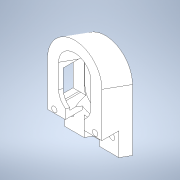
# Autodesk Inventor part: Hauptschalter
Saved by Autodesk Inventor 2021 (Build 250183000, 183)
## iProperties
Created: 2024-06-23
Part Number: Hauptschalter
Material: Generic
Document SubType Name: Modeling
Designer: Lukas
Density: 1 g/cm^3
Appearance: Default
Author: Lukas
Autodesk Inventor part; units mm, degrees
ref_plane "YZ Plane" through (0, 0, 0) normal (1, 0, 0) x (0, 1, 0)
ref_plane "XZ Plane" through (0, 0, 0) normal (0, 1, 0) x (-1, 0, 0)
ref_plane "XY Plane" through (0, 0, 0) normal (0, 0, 1) x (1, 0, 0)
sketch "Sketch1" plane through (0, 0, 0) normal (0, 0, 1) x (1, 0, 0)
  line L0 (-16, 37.209) -> (-16, 0)
  line L1 (-16, 0) -> (16, 0)
  line L2 (16, 0) -> (16, 37.209)
  arc A0 (16, 37.209) -> (-16, 37.209) centre (0, 37.209) ccw
  arc A1 (9.5, 37.209) -> (-9.5, 37.209) centre (0, 37.209) ccw
  arc A2 (-9.5, 23.375) -> (9.5, 23.375) centre (0, 23.375) ccw
  line L3 (-9.5, 23.375) -> (-9.5, 37.209)
  line L4 (9.5, 37.209) -> (9.5, 23.375)
  circle A3 centre (12, 11.493) radius 1.6
  circle A4 centre (-12, 11.493) radius 1.6
  circle A5 centre (0, 48.493) radius 1.6
  line L5 (-5, 45.2867) -> (-5, 41.2867)
  line L6 (-5, 41.2867) -> (5, 41.2867)
  line L7 (5, 41.2867) -> (5, 45.2867)
  line L8 (16, 37.209) -> (16, 53.209)
  line L9 (16, 53.209) -> (-16, 53.209)
  line L10 (-16, 53.209) -> (-16, 37.209)
  circle A6 centre (12, 18.493) radius 1.6
  circle A7 centre (-12, 18.493) radius 1.6
  point P0 (0, 0)
  point P1 (0, 0)
  point P2 (16, 18.6045)
  point P3 (0, 53.209)
  dimension "d0" = 32
  dimension "d1" = 37.209
  dimension "d2" = 13.834
  dimension "d3" = 19
  dimension "d5" = 12
  dimension "d6" = 12
  dimension "d8" = 3.2
  dimension "d26" = 10
  dimension "d27" = 4
  dimension "d34" = 37
  dimension "d35" = 11.493
  dimension "d48" = 7
  constraints: 22 end point, 8 centre point, 8 point on circle, 8 tangent, 4 equal radius, 4 horizontal alignment, 4 perpendicular, 4 vertical, 3 coincident, 3 vertical alignment, 2 midpoint, 2 parallel, 1 horizontal
  measures "d0" distance of L0.end L1.end
  measures "d1" distance of L1.end L2.end
  measures "d2" distance of L4.start L4.end
  measures "d3" distance between parallel lines of L3 L4
  measures "d5" horizontal distance of A4.centre A2.centre
  measures "d6" horizontal distance of A3.centre A2.centre
  measures "d8" diameter of A4
  measures "d26" distance of L5.end L6.end
  measures "d27" distance of L6.end L7.end
  measures "d34" vertical distance of A3.centre A5.centre
  measures "d35" distance from line of L1 A3.centre
  measures "d48" distance of A7.centre A4.centre
sketch "Sketch2" plane through (0, 0, 0) normal (1, 0, 0) x (0, 1, 0)
  line L0 (0, 0) -> (6.5515, 18)
  line L1 (0, 0) -> (19.1552, 0)
  line L2 (13.875, 0) -> (14.7849, 2.5)
  dimension "d9" = 70
  dimension "d13" = 18
  dimension "d28" = 13.875
  dimension "d31" = 2.5
  constraints: 6 end point, 1 coincident, 1 equal length, 1 horizontal, 1 parallel, 1 point on line
  measures "d9" angle of L0 L1
  measures "d13" vertical distance of L0.start L0.end
  measures "d28" distance of L2.start point (0, 0)
  measures "d31" vertical distance of L2.start L2.end
sweep "Sweep1" add profiles "Sketch1" path "Sketch2" path curves L0 contours A0 L2 L1 L0 | L10 L9 A0 | L9 L8 A0 | A3 | A4 | A5 | A6 | A7
sweep "Sweep2" add profiles "Sketch1" path "Sketch2" path curves L2 contours L4 A2 L3 A1 L5 L6 L7
extrude "Extrusion1" cut sketch "Sketch1" along normal through all contours A3 | A4 | A5 | A6 | A7
sketch "Sketch3" plane through (0, 42.7335, 18) normal (0, 0, 1) x (1, 0, 0)
  circle A0 centre (-12, -31.2405) radius 1.6 projected
  circle A1 centre (12, -31.2405) radius 1.6 projected
  circle A2 centre (-12, -31.2405) radius 3.5
  circle A3 centre (12, -31.2405) radius 3.5
  circle A4 centre (0, 5.7595) radius 3.5
  circle A5 centre (0, 5.7595) radius 1.6 projected
  line L0 (16, -36.182) -> (16, 17.027) projected
  line L1 (-16, 17.027) -> (-16, -36.182) projected
  line L2 (16, -26.182) -> (-16, -26.182)
  line L3 (-16, -26.182) -> (-16, -36.182)
  line L4 (-16, -36.182) -> (16, -36.182)
  line L5 (16, -36.182) -> (16, -26.182)
  line L6 (-16, -36.182) -> (16, -36.182) projected
  line L7 (16, -36.182) -> (-16, -36.182)
  line L8 (-16, -36.182) -> (-16, -46.182)
  line L9 (-16, -46.182) -> (16, -46.182)
  line L10 (16, -46.182) -> (16, -36.182)
  line L11 (5.5, -26.182) -> (-5.5, -26.182)
  line L12 (-5.5, -26.182) -> (-5.5, -20.182)
  line L13 (-5.5, -20.182) -> (5.5, -20.182)
  line L14 (5.5, -20.182) -> (5.5, -26.182)
  point P0 (0, -42.7335)
  point P1 (0, -20.182)
  dimension "d17" = 7
  dimension "d36" = 10
  dimension "d37" = 6
  dimension "d38" = 11
  constraints: 24 end point, 6 parallel, 3 centre point, 3 coincident, 3 horizontal, 3 perpendicular, 2 equal radius, 2 point on line, 1 collinear, 1 midpoint, 1 vertical alignment
  measures "d17" diameter of A2
  measures "d36" distance between parallel lines of L4 L2
  measures "d37" distance of L13.end L11.start
  measures "d38" distance of L12.end L13.end
extrude "Extrusion2" cut sketch "Sketch3" against normal blind 10 contours A0 | A1 | A2 | A3 | L4 L1 L2 L0 | L10 L9 L8 L4 | L2 L12 L13 L14
sketch "Sketch4" plane through (-16, 0, 0) normal (-1, 0, 0) x (0, 0, 1)
  line L0 (3, 20) -> (15.3, 20)
  line L1 (15.3, 20) -> (15.3, 39.5)
  line L2 (15.3, 39.5) -> (3, 39.5)
  line L3 (3, 39.5) -> (3, 20)
  line L4 (0, 53.209) -> (0, 0) projected
  dimension "d20" = 12.3
  dimension "d21" = 19.5
  dimension "d23" = 20
  dimension "d33" = 3
  constraints: 8 end point, 2 parallel, 1 horizontal, 1 perpendicular
  measures "d20" distance of L0.start L0.end
  measures "d21" distance of L0.end L1.end
  measures "d23" distance from line of L4.end L0
  measures "d33" distance from line of L4.end L3
extrude "Extrusion3" cut sketch "Sketch4" against normal blind 16.25
fillet "Fillet1" radius 16 2 edges at (-16, 56.4847, 9) (16, 56.4847, 9)
sketch "Sketch5" plane through (0, 42.7335, 8) normal (0, 0, 1) x (1, 0, 0)
  line L0 (-4.5, -28.3217) -> (-4.5, -33.3217)
  line L1 (-4.5, -33.3217) -> (-6, -33.3217)
  line L2 (-6, -33.3217) -> (-6, -26.5217)
  line L3 (-6, -26.5217) -> (6, -26.5217)
  line L4 (6, -26.5217) -> (6, -33.3217)
  line L5 (6, -33.3217) -> (4.5, -33.3217)
  line L6 (4.5, -33.3217) -> (4.5, -28.3217)
  line L7 (4.5, -28.3217) -> (-4.5, -28.3217)
  line L8 (16, -39.8217) -> (-16, -39.8217) projected
  line L9 (4.5, -28.3217) -> (5.5, -26.5217)
  line L10 (5.5, -24.1927) -> (5.5, -26.182) projected
  line L11 (-4.5, -28.3217) -> (-5.5, -26.5217)
  line L12 (-5.5, -26.182) -> (-5.5, -24.1927) projected
  line L13 (-4.5, -33.3217) -> (-4.5, -42.3217)
  line L14 (-4.5, -42.3217) -> (4.5, -42.3217)
  line L15 (4.5, -42.3217) -> (4.5, -33.3217)
  point P0 (0, -42.7335)
  point P1 (0, -28.3217)
  point P2 (0, -26.5217)
  point P3 (5.5, -26.5217)
  dimension "d39" = 11.5
  dimension "d40" = 1.5
  dimension "d41" = 9
  dimension "d42" = 1.8
  dimension "d43" = 5
  dimension "d49" = 9
  constraints: 22 end point, 9 perpendicular, 6 point on line, 2 midpoint, 2 vertical alignment, 1 vertical, 6 other
  measures "d39" distance between parallel lines of L8 L7
  measures "d40" distance of L4.end L5.end
  measures "d41" distance of L6.end L0.start
  measures "d42" distance between parallel lines of L3 L7
  measures "d43" distance of L5.end L6.end
  measures "d49" distance of L0.end L13.end
extrude "Extrusion6" cut sketch "Sketch5" against normal blind 5.25 contours L7 L6 L15 L8 L13 L0 | L8 L15 L14 L13
sketch "Sketch6" plane through (0, 43.7605, 18) normal (0, 0, 1) x (1, 0, 0)
  arc A0 (9.5, 0) -> (-9.5, 0) centre (0, 0) ccw projected
  ellipse E0 centre (0, -7.5783) end of major axis (0, 9.4485) minor radius 16 (16, -7.5783) -> (-16, -7.5783) ccw projected
  arc A1 (5, 7.4211) -> (-5, 7.4211) centre (0, -7.5783) ccw
  circle A2 centre (0, 4.7325) radius 1.6 projected
  circle A3 centre (0, 4.7325) radius 3.5
  line L0 (-5, 7.4211) -> (-5, 2.4211)
  line L1 (-5, 2.4211) -> (5, 2.4211)
  line L2 (5, 2.4211) -> (5, 7.4211)
  point P0 (0, -43.7605)
  dimension "d52" = 7
  dimension "d53" = 10
  dimension "d54" = 5
  constraints: 6 end point, 2 centre point, 2 coincident, 2 point on circle, 2 vertical, 1 horizontal alignment, 1 perpendicular, 1 tangent, 1 other
  measures "d52" diameter of A3
  measures "d53" distance of L0.end L1.end
  measures "d54" distance of L1.end L2.end
extrude "Extrusion7" cut sketch "Sketch6" against normal up to surface (15.5 mm away) contours L2 L1 A3 A1 | A3 L1 L0 A1 | A3 L1 picked at (-0.0643, 2.6621)
equation "\"d6\" = d5"
body "Solid1"
